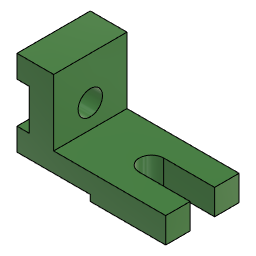
Industrial Tool 2 (Autodesk Fusion 360 design; units mm, degrees)
Autodesk Fusion 360 part; units mm, degrees
sketch "Sketch1" plane through (0, 0, 0) normal (0, 0, 1) x (1, 0, 0) in component "New Design"
  line L0 (-73, 36) -> (73, 36)
  line L1 (73, 36) -> (73, -36)
  line L2 (73, -36) -> (-73, -36)
  line L3 (-73, -36) -> (-73, 36)
  line L4 (-73, 36) -> (73, -36) construction
  line L5 (73, 36) -> (-73, -36) construction
  line L6 (-73, -36) -> (-1, -36)
  line L7 (-1, -36) -> (-1, 14)
  line L8 (-1, 14) -> (-73, 14)
  line L9 (-73, 14) -> (-73, -36)
  line L10 (23.0005, 12) -> (73, 11.9981)
  line L11 (23.0005, -12) -> (73, -11.9981)
  arc A0 (24.2094, 11.9389) -> (24.2094, -11.9389) centre (23, 0) ccw
  dimension "d1" = 146
  dimension "d2" = 72
  dimension "d3" = 72
  dimension "d4" = 50
  dimension "d5" = 24
  dimension "d6" = 50
  constraint horizontal L0
  constraint perpendicular L0 L1
  constraint parallel L0 L2
  constraint parallel L1 L3
  constraint coincident L4 origin
  constraint coincident L5 origin
  constraint horizontal L6
  constraint vertical L7
  constraint horizontal L8
  constraint vertical L9
  constraint coincident L10.start A0
  constraint coincident L1 L10.end
  constraint tangent L10 A0
  constraint coincident L11.start A0
  constraint coincident L1 L11.end
  constraint tangent L11 A0
  constraint coincident L4 A0.end
  constraint coincident L5 A0.start
  measures "d1" distance of L1.end L2.end
  measures "d2" distance of L0.end L1.end
  measures "d3" distance of L2.end L6.end
  measures "d4" distance of L2.end L8.end
  measures "d5" diameter of A0
  measures "d6" distance of L1 A0.centre
extrude "Extrude1" add sketch "Sketch1" along normal blind 25 contours L0 L1 L2 L3 L7 L8 L10 L11 A0 | L2 L3 L6 L7 L8 L9 in component "New Design"
extrude "Extrude2" cut sketch "Sketch1" along normal blind 6 contours L2 L3 L6 L7 L8 L9 in component "New Design"
sketch "Sketch2" plane through (0, 0, 25) normal (0, 0, 1) x (-1, 0, 0) in component "New Design"
  arc A0 (-23.0005, -12) -> (-23.0005, 12) centre (-23, 0) ccw
  line L0 (-23.0005, -12) -> (-73, -11.9981)
  line L1 (-73, -11.9981) -> (-73, -36)
  line L2 (-73, -36) -> (73, -36)
  line L3 (73, -36) -> (73, 36)
  line L4 (73, 36) -> (-73, 36)
  line L5 (-73, 36) -> (-73, 11.9981)
  line L6 (-73, 11.9981) -> (-23.0005, 12)
  line L7 (73, -36) -> (37, -36)
  line L8 (37, -36) -> (37, 36)
  line L9 (37, 36) -> (73, 36)
  line L10 (73, 36) -> (73, -36)
  dimension "d11" = 36
  constraint horizontal L7
  constraint vertical L8
  constraint horizontal L9
  constraint vertical L10
  constraint coincident L4 L8.end
  constraint coincident L2.end L3.start
  measures "d11" distance of L8 L10
extrude "Extrude3" add sketch "Sketch2" along normal blind 65 contours L2 L3 L4 L7 L8 L9 L10 in component "New Design"
sketch "Sketch3" plane through (-73, 0, 0) normal (-1, 0, 0) x (0, -1, 0) in component "New Design"
  line L0 (-14, 0) -> (-14, 6)
  line L1 (-14, 6) -> (36, 6)
  line L2 (36, 6) -> (36, 90)
  line L3 (36, 90) -> (-36, 90)
  line L4 (-36, 90) -> (-36, 0)
  line L5 (-36, 0) -> (-14, 0)
sketch "Sketch4" plane through (-73, 0, 45) normal (-1, 0, 0) x (0, -1, 0) in component "New Design"
  circle A0 centre (0, 3) radius 12
  circle A1 centre (0, 3) radius 30
  line L0 (-36, 45) -> (36, 45)
  line L1 (36, 45) -> (36, 21)
  line L2 (36, 21) -> (-36, 21)
  line L3 (-36, 21) -> (-36, 45)
  line L4 (36, -39) -> (-36, -39)
  line L5 (-36, -39) -> (-36, -15)
  line L6 (-36, -15) -> (36, -15)
  line L7 (36, -15) -> (36, -39)
  point P0 (0, -45)
  dimension "d14" = 24
  dimension "d15" = 60
  dimension "d16" = 48
  dimension "d17" = 24
  dimension "d18" = 24
  constraint concentric A0 A1
  constraint horizontal L0
  constraint vertical L1
  constraint horizontal L2
  constraint vertical L3
  constraint horizontal L4
  constraint vertical L5
  constraint horizontal L6
  constraint vertical L7
  measures "d14" diameter of A0
  measures "d15" diameter of A1
  measures "d16" distance of A0.centre P0
  measures "d17" distance of L0 L2
  measures "d18" distance of L4 L6
extrude "Extrude4" cut sketch "Sketch4" against normal blind 100 contours A0 in component "New Design"
sketch "Sketch5" plane through (-73, 0, 45) normal (-1, 0, 0) x (0, -1, 0) in component "New Design"
  line L0 (-24, 21) -> (-36, 21)
  line L1 (-36, 21) -> (-36, -15)
  line L2 (-36, -15) -> (-24, -15)
  line L3 (24, 21) -> (36, 21)
  line L4 (36, 21) -> (36, -15)
  line L5 (36, -15) -> (24, -15)
  constraint horizontal L0
  constraint perpendicular L0 L1
  constraint perpendicular L1 L2
  constraint horizontal L3
  constraint perpendicular L3 L4
  constraint perpendicular L4 L5
extrude "Extrude5" cut sketch "Sketch4" against normal blind 12 contours A1 L2 L6 | A1 L2 | A1 L6 in component "New Design"
sketch "Sketch6" plane through (-73, 0, 0) normal (-1, 0, 0) x (0, -1, 0) in component "New Design"
  circle A0 centre (0, 48) radius 30
  line L0 (-14, 0) -> (-14, 6)
  line L1 (-14, 6) -> (36, 6)
  line L2 (36, 6) -> (36, 90)
  line L3 (36, 90) -> (-36, 90)
  line L4 (-36, 90) -> (-36, 0)
  line L5 (-36, 0) -> (-14, 0)
  line L6 (-22.3869, 67.9706) -> (-41.8695, 67.9706)
  line L7 (-41.8695, 67.9706) -> (-41.8695, 28.0294)
  line L8 (-41.8695, 28.0294) -> (-22.3869, 28.0294)
  line L9 (-22.3869, 28.0294) -> (-22.3869, 67.9706)
  line L10 (0, 90) -> (0, 18)
  line L11 (41.8695, 28.0294) -> (22.3869, 28.0294)
  line L12 (22.3869, 28.0294) -> (22.3869, 67.9706)
  line L13 (41.8695, 67.9706) -> (41.8695, 28.0294)
  line L14 (22.3869, 67.9706) -> (41.8695, 67.9706)
  dimension "d23" = 19.4825
  constraint horizontal L6
  constraint vertical L7
  constraint horizontal L8
  constraint vertical L9
  constraint coincident A0 L6.start
  constraint midpoint L3 L10.start
  constraint coincident A0 L10.end
  constraint perpendicular L3 L10
  constraint coincident A0 L8.end
  constraint symmetric L6.start L10 L12.end
  constraint symmetric L6.end L10 L13.start
  constraint symmetric L7.end L10 L11.start
  constraint symmetric L8.end L10 L11.end
  measures "d23" distance of L6.start L6.end
extrude "Extrude6" cut sketch "Sketch6" against normal blind 12 contours A0 L2 L11 L14 | A0 L4 L6 L8 in component "New Design"
component "New Design" placed x (1, 0, 0) y (0, 1, 0) z (0, 0, 1) at (0, 0, 0)
